Autodesk Fusion 360 part; units mm, degrees
note: some values were not read from the file. Chosen so that the rebuilt part matches the saved one: which pieces of a blend or face edit are solid.
(part 2 of 4)
  circle A222 centre (-225.2664, 136.3493) radius 1.5
  circle A223 centre (-233.5214, 157.9393) radius 0.875
  circle A224 centre (-238.6014, 157.9393) radius 1.9939
  circle A225 centre (-243.6814, 157.9393) radius 0.875
  circle A226 centre (-234.7914, 155.3993) radius 1.5
  circle A227 centre (-241.1414, 152.8593) radius 1.5
  circle A228 centre (-252.5714, 157.9393) radius 0.875
  circle A229 centre (-257.6514, 157.9393) radius 1.9939
  circle A230 centre (-262.7314, 157.9393) radius 0.875
  circle A231 centre (-253.8414, 155.3993) radius 1.5
  circle A232 centre (-260.1914, 152.8593) radius 1.5
  circle A233 centre (-271.6214, 157.9393) radius 0.875
  circle A234 centre (-276.7014, 157.9393) radius 1.9939
  circle A235 centre (-281.7814, 157.9393) radius 0.875
  circle A236 centre (-272.8914, 155.3993) radius 1.5
  circle A237 centre (-279.2414, 152.8593) radius 1.5
  circle A238 centre (-290.6714, 157.9393) radius 0.875
  circle A239 centre (-295.7514, 157.9393) radius 1.9939
  circle A240 centre (-300.8314, 157.9393) radius 0.875
  circle A241 centre (-291.9414, 155.3993) radius 1.5
  circle A242 centre (-298.2914, 152.8593) radius 1.5
  arc A243 (-228.0198, 142.4254) -> (-227.3325, 143.1126) centre (-227.7593, 142.8521) ccw
  arc A244 (-228.0198, 142.4254) -> (-228.1761, 142.4693) centre (-228.176, 142.1696) ccw
  line L196 (-228.1761, 142.4693) -> (-229.0764, 142.4693)
  line L197 (-229.0764, 142.4693) -> (-229.9768, 142.4693)
  arc A245 (-229.9768, 142.4693) -> (-230.1331, 142.4254) centre (-229.9768, 142.1693) ccw
  arc A246 (-230.8204, 143.1126) -> (-230.1331, 142.4254) centre (-230.3936, 142.8521) ccw
  arc A247 (-230.8204, 143.1126) -> (-230.7764, 143.2689) centre (-231.0764, 143.2689) ccw
  line L198 (-230.7764, 143.2689) -> (-230.7764, 143.9693)
  line L199 (-230.7764, 143.9693) -> (-230.7764, 144.6696)
  arc A248 (-230.7764, 144.6696) -> (-230.8204, 144.8259) centre (-231.0764, 144.6696) ccw
  arc A249 (-230.1331, 145.5132) -> (-230.8204, 144.8259) centre (-230.3936, 145.0864) ccw
  arc A250 (-230.1331, 145.5132) -> (-229.9768, 145.4693) centre (-229.9768, 145.7693) ccw
  line L200 (-229.9768, 145.4693) -> (-229.0764, 145.4693)
  line L201 (-229.0764, 145.4693) -> (-228.1761, 145.4693)
  arc A251 (-228.1761, 145.4693) -> (-228.0198, 145.5132) centre (-228.1761, 145.7693) ccw
  arc A252 (-227.3325, 144.8259) -> (-228.0198, 145.5132) centre (-227.7593, 145.0864) ccw
  arc A253 (-227.3325, 144.8259) -> (-227.3764, 144.6696) centre (-227.0764, 144.6696) ccw
  line L202 (-227.3764, 144.6696) -> (-227.3764, 143.9693)
  line L203 (-227.3764, 143.9693) -> (-227.3764, 143.2689)
  arc A254 (-227.3764, 143.2689) -> (-227.3325, 143.1126) centre (-227.0764, 143.2689) ccw
  circle A255 centre (-229.0764, 138.8893) radius 1.9939
  circle A256 centre (-234.1564, 138.8893) radius 0.875
  circle A257 centre (-243.0464, 138.8893) radius 0.875
  arc A258 (-247.0698, 142.4254) -> (-246.3825, 143.1126) centre (-246.8093, 142.8521) ccw
  arc A259 (-247.0698, 142.4254) -> (-247.2261, 142.4693) centre (-247.226, 142.1696) ccw
  line L204 (-247.2261, 142.4693) -> (-248.1264, 142.4693)
  line L205 (-248.1264, 142.4693) -> (-249.0268, 142.4693)
  arc A260 (-249.0268, 142.4693) -> (-249.1831, 142.4254) centre (-249.0268, 142.1693) ccw
  arc A261 (-249.8704, 143.1126) -> (-249.1831, 142.4254) centre (-249.4436, 142.8521) ccw
  arc A262 (-249.8704, 143.1126) -> (-249.8264, 143.2689) centre (-250.1264, 143.2689) ccw
  line L206 (-249.8264, 143.2689) -> (-249.8264, 143.9693)
  line L207 (-249.8264, 143.9693) -> (-249.8264, 144.6696)
  arc A263 (-249.8264, 144.6696) -> (-249.8704, 144.8259) centre (-250.1264, 144.6696) ccw
  arc A264 (-249.1831, 145.5132) -> (-249.8704, 144.8259) centre (-249.4436, 145.0864) ccw
  arc A265 (-249.1831, 145.5132) -> (-249.0268, 145.4693) centre (-249.0268, 145.7693) ccw
  line L208 (-249.0268, 145.4693) -> (-248.1264, 145.4693)
  line L209 (-248.1264, 145.4693) -> (-247.2261, 145.4693)
  arc A266 (-247.2261, 145.4693) -> (-247.0698, 145.5132) centre (-247.2261, 145.7693) ccw
  arc A267 (-246.3825, 144.8259) -> (-247.0698, 145.5132) centre (-246.8093, 145.0864) ccw
  arc A268 (-246.3825, 144.8259) -> (-246.4264, 144.6696) centre (-246.1264, 144.6696) ccw
  line L210 (-246.4264, 144.6696) -> (-246.4264, 143.9693)
  line L211 (-246.4264, 143.9693) -> (-246.4264, 143.2689)
  arc A269 (-246.4264, 143.2689) -> (-246.3825, 143.1126) centre (-246.1264, 143.2689) ccw
  circle A270 centre (-248.1264, 138.8893) radius 1.9939
  circle A271 centre (-253.2064, 138.8893) radius 0.875
  circle A272 centre (-262.0964, 138.8893) radius 0.875
  circle A273 centre (-231.6164, 133.8093) radius 1.5
  circle A274 centre (-244.3164, 136.3493) radius 1.5
  circle A275 centre (-250.6664, 133.8093) radius 1.5
  circle A276 centre (-263.3664, 136.3493) radius 1.5
  arc A277 (-266.1198, 142.4254) -> (-265.4325, 143.1126) centre (-265.8593, 142.8521) ccw
  arc A278 (-266.1198, 142.4254) -> (-266.2761, 142.4693) centre (-266.276, 142.1696) ccw
  line L212 (-266.2761, 142.4693) -> (-267.1764, 142.4693)
  line L213 (-267.1764, 142.4693) -> (-268.0768, 142.4693)
  arc A279 (-268.0768, 142.4693) -> (-268.2331, 142.4254) centre (-268.0768, 142.1693) ccw
  arc A280 (-268.9204, 143.1126) -> (-268.2331, 142.4254) centre (-268.4936, 142.8521) ccw
  arc A281 (-268.9204, 143.1126) -> (-268.8764, 143.2689) centre (-269.1764, 143.2689) ccw
  line L214 (-268.8764, 143.2689) -> (-268.8764, 143.9693)
  line L215 (-268.8764, 143.9693) -> (-268.8764, 144.6696)
  arc A282 (-268.8764, 144.6696) -> (-268.9204, 144.8259) centre (-269.1764, 144.6696) ccw
  arc A283 (-268.2331, 145.5132) -> (-268.9204, 144.8259) centre (-268.4936, 145.0864) ccw
  arc A284 (-268.2331, 145.5132) -> (-268.0768, 145.4693) centre (-268.0768, 145.7693) ccw
  line L216 (-268.0768, 145.4693) -> (-267.1764, 145.4693)
  line L217 (-267.1764, 145.4693) -> (-266.2761, 145.4693)
  arc A285 (-266.2761, 145.4693) -> (-266.1198, 145.5132) centre (-266.2761, 145.7693) ccw
  arc A286 (-265.4325, 144.8259) -> (-266.1198, 145.5132) centre (-265.8593, 145.0864) ccw
  arc A287 (-265.4325, 144.8259) -> (-265.4764, 144.6696) centre (-265.1764, 144.6696) ccw
  line L218 (-265.4764, 144.6696) -> (-265.4764, 143.9693)
  line L219 (-265.4764, 143.9693) -> (-265.4764, 143.2689)
  arc A288 (-265.4764, 143.2689) -> (-265.4325, 143.1126) centre (-265.1764, 143.2689) ccw
  circle A289 centre (-267.1764, 138.8893) radius 1.9939
  circle A290 centre (-272.2564, 138.8893) radius 0.875
  circle A291 centre (-281.1464, 138.8893) radius 0.875
  arc A292 (-287.9704, 143.1126) -> (-287.2831, 142.4254) centre (-287.5436, 142.8521) ccw
  arc A293 (-287.9704, 143.1126) -> (-287.9264, 143.2689) centre (-288.2264, 143.2689) ccw
  line L220 (-287.9264, 143.2689) -> (-287.9264, 143.9693)
  line L221 (-287.9264, 143.9693) -> (-287.9264, 144.6696)
  arc A294 (-287.9264, 144.6696) -> (-287.9704, 144.8259) centre (-288.2264, 144.6696) ccw
  arc A295 (-287.2831, 145.5132) -> (-287.9704, 144.8259) centre (-287.5436, 145.0864) ccw
  arc A296 (-287.2831, 145.5132) -> (-287.1268, 145.4693) centre (-287.1268, 145.7693) ccw
  line L222 (-287.1268, 145.4693) -> (-286.2264, 145.4693)
  line L223 (-286.2264, 145.4693) -> (-285.3261, 145.4693)
  arc A297 (-285.3261, 145.4693) -> (-285.1698, 145.5132) centre (-285.3261, 145.7693) ccw
  arc A298 (-284.4825, 144.8259) -> (-285.1698, 145.5132) centre (-284.9093, 145.0864) ccw
  arc A299 (-284.4825, 144.8259) -> (-284.5264, 144.6696) centre (-284.2264, 144.6696) ccw
  line L224 (-284.5264, 144.6696) -> (-284.5264, 143.9693)
  line L225 (-284.5264, 143.9693) -> (-284.5264, 143.2689)
  arc A300 (-284.5264, 143.2689) -> (-284.4825, 143.1126) centre (-284.2264, 143.2689) ccw
  arc A301 (-285.1698, 142.4254) -> (-284.4825, 143.1126) centre (-284.9093, 142.8521) ccw
  arc A302 (-285.1698, 142.4254) -> (-285.3261, 142.4693) centre (-285.326, 142.1696) ccw
  line L226 (-285.3261, 142.4693) -> (-286.2264, 142.4693)
  line L227 (-286.2264, 142.4693) -> (-287.1268, 142.4693)
  arc A303 (-287.1268, 142.4693) -> (-287.2831, 142.4254) centre (-287.1268, 142.1693) ccw
  arc A304 (-307.0204, 143.1126) -> (-306.3331, 142.4254) centre (-306.5936, 142.8521) ccw
  arc A305 (-307.0204, 143.1126) -> (-306.9764, 143.2689) centre (-307.2764, 143.2689) ccw
  line L228 (-306.9764, 143.2689) -> (-306.9764, 143.9693)
  line L229 (-306.9764, 143.9693) -> (-306.9764, 144.6696)
  arc A306 (-306.9764, 144.6696) -> (-307.0204, 144.8259) centre (-307.2764, 144.6696) ccw
  arc A307 (-306.3331, 145.5132) -> (-307.0204, 144.8259) centre (-306.5936, 145.0864) ccw
  arc A308 (-306.3331, 145.5132) -> (-306.1768, 145.4693) centre (-306.1768, 145.7693) ccw
  line L230 (-306.1768, 145.4693) -> (-305.2764, 145.4693)
  line L231 (-305.2764, 145.4693) -> (-304.3761, 145.4693)
  arc A309 (-304.3761, 145.4693) -> (-304.2198, 145.5132) centre (-304.3761, 145.7693) ccw
  arc A310 (-303.5325, 144.8259) -> (-304.2198, 145.5132) centre (-303.9593, 145.0864) ccw
  arc A311 (-303.5325, 144.8259) -> (-303.5764, 144.6696) centre (-303.2764, 144.6696) ccw
  line L232 (-303.5764, 144.6696) -> (-303.5764, 143.9693)
  line L233 (-303.5764, 143.9693) -> (-303.5764, 143.2689)
  arc A312 (-303.5764, 143.2689) -> (-303.5325, 143.1126) centre (-303.2764, 143.2689) ccw
  arc A313 (-304.2198, 142.4254) -> (-303.5325, 143.1126) centre (-303.9593, 142.8521) ccw
  arc A314 (-304.2198, 142.4254) -> (-304.3761, 142.4693) centre (-304.376, 142.1696) ccw
  line L234 (-304.3761, 142.4693) -> (-305.2764, 142.4693)
  line L235 (-305.2764, 142.4693) -> (-306.1768, 142.4693)
  arc A315 (-306.1768, 142.4693) -> (-306.3331, 142.4254) centre (-306.1768, 142.1693) ccw
  circle A316 centre (-286.2264, 138.8893) radius 1.9939
  circle A317 centre (-291.3064, 138.8893) radius 0.875
  circle A318 centre (-300.1964, 138.8893) radius 0.875
  circle A319 centre (-305.2764, 138.8893) radius 1.9939
  circle A320 centre (-269.7164, 133.8093) radius 1.5
  circle A321 centre (-282.4164, 136.3493) radius 1.5
  circle A322 centre (-288.7664, 133.8093) radius 1.5
  circle A323 centre (-301.4664, 136.3493) radius 1.5
  circle A324 centre (-326.7077, 191.2768) radius 1.1
  circle A325 centre (-343.0589, 176.9893) radius 0.875
  arc A326 (-349.8829, 181.2126) -> (-349.1956, 180.5254) centre (-349.4561, 180.9521) ccw
  arc A327 (-349.8829, 181.2126) -> (-349.8389, 181.3689) centre (-350.1389, 181.3689) ccw
  line L236 (-349.8389, 181.3689) -> (-349.8389, 182.0693)
  line L237 (-349.8389, 182.0693) -> (-349.8389, 182.7696)
  arc A328 (-349.8389, 182.7696) -> (-349.8829, 182.9259) centre (-350.1389, 182.7696) ccw
  arc A329 (-349.1956, 183.6132) -> (-349.8829, 182.9259) centre (-349.4561, 183.1864) ccw
  arc A330 (-349.1956, 183.6132) -> (-349.0393, 183.5693) centre (-349.0393, 183.8693) ccw
  line L238 (-349.0393, 183.5693) -> (-348.1389, 183.5693)
  line L239 (-348.1389, 183.5693) -> (-347.2386, 183.5693)
  arc A331 (-347.2386, 183.5693) -> (-347.0823, 183.6132) centre (-347.2386, 183.8693) ccw
  arc A332 (-346.395, 182.9259) -> (-347.0823, 183.6132) centre (-346.8218, 183.1864) ccw
  arc A333 (-346.395, 182.9259) -> (-346.4389, 182.7696) centre (-346.1389, 182.7696) ccw
  line L240 (-346.4389, 182.7696) -> (-346.4389, 182.0693)
  line L241 (-346.4389, 182.0693) -> (-346.4389, 181.3689)
  arc A334 (-346.4389, 181.3689) -> (-346.395, 181.2126) centre (-346.1389, 181.3689) ccw
  arc A335 (-347.0823, 180.5254) -> (-346.395, 181.2126) centre (-346.8218, 180.9521) ccw
  arc A336 (-347.0823, 180.5254) -> (-347.2386, 180.5693) centre (-347.2385, 180.2696) ccw
  line L242 (-347.2386, 180.5693) -> (-348.1389, 180.5693)
  line L243 (-348.1389, 180.5693) -> (-349.0393, 180.5693)
  arc A337 (-349.0393, 180.5693) -> (-349.1956, 180.5254) centre (-349.0393, 180.2693) ccw
  circle A338 centre (-348.1389, 176.9893) radius 1.9939
  circle A339 centre (-353.2189, 176.9893) radius 0.875
  circle A340 centre (-362.1089, 176.9893) radius 0.875
  arc A341 (-368.9329, 181.2126) -> (-368.2456, 180.5254) centre (-368.5061, 180.9521) ccw
  arc A342 (-368.9329, 181.2126) -> (-368.8889, 181.3689) centre (-369.1889, 181.3689) ccw
  line L244 (-368.8889, 181.3689) -> (-368.8889, 182.0693)
  line L245 (-368.8889, 182.0693) -> (-368.8889, 182.7696)
  arc A343 (-368.8889, 182.7696) -> (-368.9329, 182.9259) centre (-369.1889, 182.7696) ccw
  arc A344 (-368.2456, 183.6132) -> (-368.9329, 182.9259) centre (-368.5061, 183.1864) ccw
  arc A345 (-368.2456, 183.6132) -> (-368.0893, 183.5693) centre (-368.0893, 183.8693) ccw
  line L246 (-368.0893, 183.5693) -> (-367.1889, 183.5693)
  line L247 (-367.1889, 183.5693) -> (-366.2886, 183.5693)
  arc A346 (-366.2886, 183.5693) -> (-366.1323, 183.6132) centre (-366.2886, 183.8693) ccw
  arc A347 (-365.445, 182.9259) -> (-366.1323, 183.6132) centre (-365.8718, 183.1864) ccw
  arc A348 (-365.445, 182.9259) -> (-365.4889, 182.7696) centre (-365.1889, 182.7696) ccw
  line L248 (-365.4889, 182.7696) -> (-365.4889, 182.0693)
  line L249 (-365.4889, 182.0693) -> (-365.4889, 181.3689)
  arc A349 (-365.4889, 181.3689) -> (-365.445, 181.2126) centre (-365.1889, 181.3689) ccw
  arc A350 (-366.1323, 180.5254) -> (-365.445, 181.2126) centre (-365.8718, 180.9521) ccw
  arc A351 (-366.1323, 180.5254) -> (-366.2886, 180.5693) centre (-366.2885, 180.2696) ccw
  line L250 (-366.2886, 180.5693) -> (-367.1889, 180.5693)
  line L251 (-367.1889, 180.5693) -> (-368.0893, 180.5693)
  arc A352 (-368.0893, 180.5693) -> (-368.2456, 180.5254) centre (-368.0893, 180.2693) ccw
  circle A353 centre (-367.1889, 176.9893) radius 1.9939
  circle A354 centre (-372.2689, 176.9893) radius 0.875
  circle A355 centre (-381.1589, 176.9893) radius 0.875
  circle A356 centre (-344.3289, 174.4493) radius 1.5
  arc A357 (-316.5454, 162.1626) -> (-315.8581, 161.4754) centre (-316.1186, 161.9021) ccw
  arc A358 (-316.5454, 162.1626) -> (-316.5014, 162.3189) centre (-316.8014, 162.3189) ccw
  line L252 (-316.5014, 162.3189) -> (-316.5014, 163.0193)
  line L253 (-316.5014, 163.0193) -> (-316.5014, 163.7196)
  arc A359 (-316.5014, 163.7196) -> (-316.5454, 163.8759) centre (-316.8014, 163.7196) ccw
  arc A360 (-315.8581, 164.5632) -> (-316.5454, 163.8759) centre (-316.1186, 164.1364) ccw
  arc A361 (-315.8581, 164.5632) -> (-315.7018, 164.5193) centre (-315.7018, 164.8193) ccw
  line L254 (-315.7018, 164.5193) -> (-314.8014, 164.5193)
  line L255 (-314.8014, 164.5193) -> (-313.9011, 164.5193)
  arc A362 (-313.9011, 164.5193) -> (-313.7448, 164.5632) centre (-313.9011, 164.8193) ccw
  arc A363 (-313.0575, 163.8759) -> (-313.7448, 164.5632) centre (-313.4843, 164.1364) ccw
  arc A364 (-313.0575, 163.8759) -> (-313.1014, 163.7196) centre (-312.8014, 163.7196) ccw
  line L256 (-313.1014, 163.7196) -> (-313.1014, 163.0193)
  line L257 (-313.1014, 163.0193) -> (-313.1014, 162.3189)
  arc A365 (-313.1014, 162.3189) -> (-313.0575, 162.1626) centre (-312.8014, 162.3189) ccw
  arc A366 (-313.7448, 161.4754) -> (-313.0575, 162.1626) centre (-313.4843, 161.9021) ccw
  arc A367 (-313.7448, 161.4754) -> (-313.9011, 161.5193) centre (-313.901, 161.2196) ccw
  line L258 (-313.9011, 161.5193) -> (-314.8014, 161.5193)
  line L259 (-314.8014, 161.5193) -> (-315.7018, 161.5193)
  arc A368 (-315.7018, 161.5193) -> (-315.8581, 161.4754) centre (-315.7018, 161.2193) ccw
  arc A369 (-335.5954, 162.1626) -> (-334.9081, 161.4754) centre (-335.1686, 161.9021) ccw
  arc A370 (-335.5954, 162.1626) -> (-335.5514, 162.3189) centre (-335.8514, 162.3189) ccw
  line L260 (-335.5514, 162.3189) -> (-335.5514, 163.0193)
  line L261 (-335.5514, 163.0193) -> (-335.5514, 163.7196)
  arc A371 (-335.5514, 163.7196) -> (-335.5954, 163.8759) centre (-335.8514, 163.7196) ccw
  arc A372 (-334.9081, 164.5632) -> (-335.5954, 163.8759) centre (-335.1686, 164.1364) ccw
  arc A373 (-334.9081, 164.5632) -> (-334.7518, 164.5193) centre (-334.7518, 164.8193) ccw
  line L262 (-334.7518, 164.5193) -> (-333.8514, 164.5193)
  line L263 (-333.8514, 164.5193) -> (-332.9511, 164.5193)
  arc A374 (-332.9511, 164.5193) -> (-332.7948, 164.5632) centre (-332.9511, 164.8193) ccw
  arc A375 (-332.1075, 163.8759) -> (-332.7948, 164.5632) centre (-332.5343, 164.1364) ccw
  arc A376 (-332.1075, 163.8759) -> (-332.1514, 163.7196) centre (-331.8514, 163.7196) ccw
  line L264 (-332.1514, 163.7196) -> (-332.1514, 163.0193)
  line L265 (-332.1514, 163.0193) -> (-332.1514, 162.3189)
  arc A377 (-332.1514, 162.3189) -> (-332.1075, 162.1626) centre (-331.8514, 162.3189) ccw
  arc A378 (-332.7948, 161.4754) -> (-332.1075, 162.1626) centre (-332.5343, 161.9021) ccw
  arc A379 (-332.7948, 161.4754) -> (-332.9511, 161.5193) centre (-332.951, 161.2196) ccw
  line L266 (-332.9511, 161.5193) -> (-333.8514, 161.5193)
  line L267 (-333.8514, 161.5193) -> (-334.7518, 161.5193)
  arc A380 (-334.7518, 161.5193) -> (-334.9081, 161.4754) centre (-334.7518, 161.2193) ccw
  circle A381 centre (-363.3789, 174.4493) radius 1.5
  circle A382 centre (-350.6789, 171.9093) radius 1.5
  circle A383 centre (-382.4289, 174.4493) radius 1.5
  circle A384 centre (-369.7289, 171.9093) radius 1.5
  arc A385 (-354.6454, 162.1626) -> (-353.9581, 161.4754) centre (-354.2186, 161.9021) ccw
  arc A386 (-354.6454, 162.1626) -> (-354.6014, 162.3189) centre (-354.9014, 162.3189) ccw
  line L268 (-354.6014, 162.3189) -> (-354.6014, 163.0193)
  line L269 (-354.6014, 163.0193) -> (-354.6014, 163.7196)
  arc A387 (-354.6014, 163.7196) -> (-354.6454, 163.8759) centre (-354.9014, 163.7196) ccw
  arc A388 (-353.9581, 164.5632) -> (-354.6454, 163.8759) centre (-354.2186, 164.1364) ccw
  arc A389 (-353.9581, 164.5632) -> (-353.8018, 164.5193) centre (-353.8018, 164.8193) ccw
  line L270 (-353.8018, 164.5193) -> (-352.9014, 164.5193)
  line L271 (-352.9014, 164.5193) -> (-352.0011, 164.5193)
  arc A390 (-352.0011, 164.5193) -> (-351.8448, 164.5632) centre (-352.0011, 164.8193) ccw
  arc A391 (-351.1575, 163.8759) -> (-351.8448, 164.5632) centre (-351.5843, 164.1364) ccw
  arc A392 (-351.1575, 163.8759) -> (-351.2014, 163.7196) centre (-350.9014, 163.7196) ccw
  line L272 (-351.2014, 163.7196) -> (-351.2014, 163.0193)
  line L273 (-351.2014, 163.0193) -> (-351.2014, 162.3189)
  arc A393 (-351.2014, 162.3189) -> (-351.1575, 162.1626) centre (-350.9014, 162.3189) ccw
  arc A394 (-351.8448, 161.4754) -> (-351.1575, 162.1626) centre (-351.5843, 161.9021) ccw
  arc A395 (-351.8448, 161.4754) -> (-352.0011, 161.5193) centre (-352.001, 161.2196) ccw
  line L274 (-352.0011, 161.5193) -> (-352.9014, 161.5193)
  line L275 (-352.9014, 161.5193) -> (-353.8018, 161.5193)
  arc A396 (-353.8018, 161.5193) -> (-353.9581, 161.4754) centre (-353.8018, 161.2193) ccw
  arc A397 (-373.6954, 162.1626) -> (-373.0081, 161.4754) centre (-373.2686, 161.9021) ccw
  arc A398 (-373.6954, 162.1626) -> (-373.6514, 162.3189) centre (-373.9514, 162.3189) ccw
  line L276 (-373.6514, 162.3189) -> (-373.6514, 163.0193)
  line L277 (-373.6514, 163.0193) -> (-373.6514, 163.7196)
  arc A399 (-373.6514, 163.7196) -> (-373.6954, 163.8759) centre (-373.9514, 163.7196) ccw
  arc A400 (-373.0081, 164.5632) -> (-373.6954, 163.8759) centre (-373.2686, 164.1364) ccw
  arc A401 (-373.0081, 164.5632) -> (-372.8518, 164.5193) centre (-372.8518, 164.8193) ccw
  line L278 (-372.8518, 164.5193) -> (-371.9514, 164.5193)
  line L279 (-371.9514, 164.5193) -> (-371.0511, 164.5193)
  arc A402 (-371.0511, 164.5193) -> (-370.8948, 164.5632) centre (-371.0511, 164.8193) ccw
  arc A403 (-370.2075, 163.8759) -> (-370.8948, 164.5632) centre (-370.6343, 164.1364) ccw
  arc A404 (-370.2075, 163.8759) -> (-370.2514, 163.7196) centre (-369.9514, 163.7196) ccw
  line L280 (-370.2514, 163.7196) -> (-370.2514, 163.0193)
  line L281 (-370.2514, 163.0193) -> (-370.2514, 162.3189)
  arc A405 (-370.2514, 162.3189) -> (-370.2075, 162.1626) centre (-369.9514, 162.3189) ccw
  arc A406 (-370.8948, 161.4754) -> (-370.2075, 162.1626) centre (-370.6343, 161.9021) ccw
  arc A407 (-370.8948, 161.4754) -> (-371.0511, 161.5193) centre (-371.051, 161.2196) ccw
  line L282 (-371.0511, 161.5193) -> (-371.9514, 161.5193)
  line L283 (-371.9514, 161.5193) -> (-372.8518, 161.5193)
  arc A408 (-372.8518, 161.5193) -> (-373.0081, 161.4754) centre (-372.8518, 161.2193) ccw
  arc A409 (-411.7954, 185.9751) -> (-411.1081, 185.2879) centre (-411.3686, 185.7146) ccw
  arc A410 (-411.7954, 185.9751) -> (-411.7514, 186.1314) centre (-412.0514, 186.1314) ccw
  line L284 (-411.7514, 186.1314) -> (-411.7514, 186.8318)
  line L285 (-411.7514, 186.8318) -> (-411.7514, 187.5321)
  arc A411 (-411.7514, 187.5321) -> (-411.7954, 187.6884) centre (-412.0514, 187.5321) ccw
  arc A412 (-411.1081, 188.3757) -> (-411.7954, 187.6884) centre (-411.3686, 187.9489) ccw
  arc A413 (-411.1081, 188.3757) -> (-410.9518, 188.3318) centre (-410.9518, 188.6318) ccw
  line L286 (-410.9518, 188.3318) -> (-410.0514, 188.3318)
  line L287 (-410.0514, 188.3318) -> (-409.1511, 188.3318)
  arc A414 (-409.1511, 188.3318) -> (-408.9948, 188.3757) centre (-409.1511, 188.6318) ccw
  arc A415 (-408.3075, 187.6884) -> (-408.9948, 188.3757) centre (-408.7343, 187.9489) ccw
  arc A416 (-408.3075, 187.6884) -> (-408.3514, 187.5321) centre (-408.0514, 187.5321) ccw
  line L288 (-408.3514, 187.5321) -> (-408.3514, 186.8318)
  line L289 (-408.3514, 186.8318) -> (-408.3514, 186.1314)
  arc A417 (-408.3514, 186.1314) -> (-408.3075, 185.9751) centre (-408.0514, 186.1314) ccw
  arc A418 (-408.9948, 185.2879) -> (-408.3075, 185.9751) centre (-408.7343, 185.7146) ccw
  arc A419 (-408.9948, 185.2879) -> (-409.1511, 185.3318) centre (-409.151, 185.0321) ccw
  line L290 (-409.1511, 185.3318) -> (-410.0514, 185.3318)
  line L291 (-410.0514, 185.3318) -> (-410.9518, 185.3318)
  arc A420 (-410.9518, 185.3318) -> (-411.1081, 185.2879) centre (-410.9518, 185.0318) ccw
  arc A421 (-387.9829, 181.2126) -> (-387.2956, 180.5254) centre (-387.5561, 180.9521) ccw
  arc A422 (-387.9829, 181.2126) -> (-387.9389, 181.3689) centre (-388.2389, 181.3689) ccw
  line L292 (-387.9389, 181.3689) -> (-387.9389, 182.0693)
  line L293 (-387.9389, 182.0693) -> (-387.9389, 182.7696)
  arc A423 (-387.9389, 182.7696) -> (-387.9829, 182.9259) centre (-388.2389, 182.7696) ccw
  arc A424 (-387.2956, 183.6132) -> (-387.9829, 182.9259) centre (-387.5561, 183.1864) ccw
  arc A425 (-387.2956, 183.6132) -> (-387.1393, 183.5693) centre (-387.1393, 183.8693) ccw
  line L294 (-387.1393, 183.5693) -> (-386.2389, 183.5693)
  line L295 (-386.2389, 183.5693) -> (-385.3386, 183.5693)
  arc A426 (-385.3386, 183.5693) -> (-385.1823, 183.6132) centre (-385.3386, 183.8693) ccw
  arc A427 (-384.495, 182.9259) -> (-385.1823, 183.6132) centre (-384.9218, 183.1864) ccw
  arc A428 (-384.495, 182.9259) -> (-384.5389, 182.7696) centre (-384.2389, 182.7696) ccw
  line L296 (-384.5389, 182.7696) -> (-384.5389, 182.0693)
  line L297 (-384.5389, 182.0693) -> (-384.5389, 181.3689)
  arc A429 (-384.5389, 181.3689) -> (-384.495, 181.2126) centre (-384.2389, 181.3689) ccw
  arc A430 (-385.1823, 180.5254) -> (-384.495, 181.2126) centre (-384.9218, 180.9521) ccw
  arc A431 (-385.1823, 180.5254) -> (-385.3386, 180.5693) centre (-385.3385, 180.2696) ccw
  line L298 (-385.3386, 180.5693) -> (-386.2389, 180.5693)
  line L299 (-386.2389, 180.5693) -> (-387.1393, 180.5693)
  arc A432 (-387.1393, 180.5693) -> (-387.2956, 180.5254) centre (-387.1393, 180.2693) ccw
  circle A433 centre (-386.2389, 176.9893) radius 1.9939
  circle A434 centre (-391.3189, 176.9893) radius 0.875
  circle A435 centre (-404.9714, 181.7518) radius 0.875
  circle A436 centre (-410.0514, 181.7518) radius 1.9939
  circle A437 centre (-415.1314, 181.7518) radius 0.875
  circle A438 centre (-406.2414, 179.2118) radius 1.5
  circle A439 centre (-412.5914, 176.6718) radius 1.5
  arc A440 (-430.8454, 185.9751) -> (-430.1581, 185.2879) centre (-430.4186, 185.7146) ccw
  arc A441 (-430.8454, 185.9751) -> (-430.8014, 186.1314) centre (-431.1014, 186.1314) ccw
  line L300 (-430.8014, 186.1314) -> (-430.8014, 186.8318)
  line L301 (-430.8014, 186.8318) -> (-430.8014, 187.5321)
  arc A442 (-430.8014, 187.5321) -> (-430.8454, 187.6884) centre (-431.1014, 187.5321) ccw
  arc A443 (-430.1581, 188.3757) -> (-430.8454, 187.6884) centre (-430.4186, 187.9489) ccw
  arc A444 (-430.1581, 188.3757) -> (-430.0018, 188.3318) centre (-430.0018, 188.6318) ccw
  line L302 (-430.0018, 188.3318) -> (-429.1014, 188.3318)
  line L303 (-429.1014, 188.3318) -> (-428.2011, 188.3318)
  arc A445 (-428.2011, 188.3318) -> (-428.0448, 188.3757) centre (-428.2011, 188.6318) ccw
  arc A446 (-427.3575, 187.6884) -> (-428.0448, 188.3757) centre (-427.7843, 187.9489) ccw
  arc A447 (-427.3575, 187.6884) -> (-427.4014, 187.5321) centre (-427.1014, 187.5321) ccw
  line L304 (-427.4014, 187.5321) -> (-427.4014, 186.8318)
  line L305 (-427.4014, 186.8318) -> (-427.4014, 186.1314)
  arc A448 (-427.4014, 186.1314) -> (-427.3575, 185.9751) centre (-427.1014, 186.1314) ccw
  arc A449 (-428.0448, 185.2879) -> (-427.3575, 185.9751) centre (-427.7843, 185.7146) ccw
  arc A450 (-428.0448, 185.2879) -> (-428.2011, 185.3318) centre (-428.201, 185.0321) ccw
  line L306 (-428.2011, 185.3318) -> (-429.1014, 185.3318)
  line L307 (-429.1014, 185.3318) -> (-430.0018, 185.3318)
  arc A451 (-430.0018, 185.3318) -> (-430.1581, 185.2879) centre (-430.0018, 185.0318) ccw
  circle A452 centre (-462.4389, 191.2768) radius 1.1
  arc A453 (-449.8954, 185.9751) -> (-449.2081, 185.2879) centre (-449.4686, 185.7146) ccw
  arc A454 (-449.8954, 185.9751) -> (-449.8514, 186.1314) centre (-450.1514, 186.1314) ccw
  line L308 (-449.8514, 186.1314) -> (-449.8514, 186.8318)
  line L309 (-449.8514, 186.8318) -> (-449.8514, 187.5321)
  arc A455 (-449.8514, 187.5321) -> (-449.8954, 187.6884) centre (-450.1514, 187.5321) ccw
  arc A456 (-449.2081, 188.3757) -> (-449.8954, 187.6884) centre (-449.4686, 187.9489) ccw
  arc A457 (-449.2081, 188.3757) -> (-449.0518, 188.3318) centre (-449.0518, 188.6318) ccw
  line L310 (-449.0518, 188.3318) -> (-448.1514, 188.3318)
  line L311 (-448.1514, 188.3318) -> (-447.2511, 188.3318)
  arc A458 (-447.2511, 188.3318) -> (-447.0948, 188.3757) centre (-447.2511, 188.6318) ccw
  arc A459 (-446.4075, 187.6884) -> (-447.0948, 188.3757) centre (-446.8343, 187.9489) ccw
  arc A460 (-446.4075, 187.6884) -> (-446.4514, 187.5321) centre (-446.1514, 187.5321) ccw
  line L312 (-446.4514, 187.5321) -> (-446.4514, 186.8318)
  line L313 (-446.4514, 186.8318) -> (-446.4514, 186.1314)
  arc A461 (-446.4514, 186.1314) -> (-446.4075, 185.9751) centre (-446.1514, 186.1314) ccw
  arc A462 (-447.0948, 185.2879) -> (-446.4075, 185.9751) centre (-446.8343, 185.7146) ccw
  arc A463 (-447.0948, 185.2879) -> (-447.2511, 185.3318) centre (-447.251, 185.0321) ccw
  line L314 (-447.2511, 185.3318) -> (-448.1514, 185.3318)
  line L315 (-448.1514, 185.3318) -> (-449.0518, 185.3318)
  arc A464 (-449.0518, 185.3318) -> (-449.2081, 185.2879) centre (-449.0518, 185.0318) ccw
  circle A465 centre (-424.0214, 181.7518) radius 0.875
  circle A466 centre (-429.1014, 181.7518) radius 1.9939
  circle A467 centre (-434.1814, 181.7518) radius 0.875
  circle A468 centre (-443.0714, 181.7518) radius 0.875
  circle A469 centre (-425.2914, 179.2118) radius 1.5
  circle A470 centre (-431.6414, 176.6718) radius 1.5
  circle A471 centre (-448.1514, 181.7518) radius 1.9939
  circle A472 centre (-453.2314, 181.7518) radius 0.875
  circle A473 centre (-444.3414, 179.2118) radius 1.5
  circle A474 centre (-450.6914, 176.6718) radius 1.5
  circle A475 centre (-388.7789, 171.9093) radius 1.5
  arc A476 (-399.5454, 162.1626) -> (-398.8581, 161.4754) centre (-399.1186, 161.9021) ccw
  arc A477 (-399.5454, 162.1626) -> (-399.5014, 162.3189) centre (-399.8014, 162.3189) ccw
  line L316 (-399.5014, 162.3189) -> (-399.5014, 163.0193)
  line L317 (-399.5014, 163.0193) -> (-399.5014, 163.7196)
  arc A478 (-399.5014, 163.7196) -> (-399.5454, 163.8759) centre (-399.8014, 163.7196) ccw
  arc A479 (-398.8581, 164.5632) -> (-399.5454, 163.8759) centre (-399.1186, 164.1364) ccw
  arc A480 (-398.8581, 164.5632) -> (-398.7018, 164.5193) centre (-398.7018, 164.8193) ccw
  line L318 (-398.7018, 164.5193) -> (-397.8014, 164.5193)
  line L319 (-397.8014, 164.5193) -> (-396.9011, 164.5193)
  arc A481 (-396.9011, 164.5193) -> (-396.7448, 164.5632) centre (-396.9011, 164.8193) ccw
  arc A482 (-396.0575, 163.8759) -> (-396.7448, 164.5632) centre (-396.4843, 164.1364) ccw
  arc A483 (-396.0575, 163.8759) -> (-396.1014, 163.7196) centre (-395.8014, 163.7196) ccw
  line L320 (-396.1014, 163.7196) -> (-396.1014, 163.0193)
  line L321 (-396.1014, 163.0193) -> (-396.1014, 162.3189)
  arc A484 (-396.1014, 162.3189) -> (-396.0575, 162.1626) centre (-395.8014, 162.3189) ccw
  arc A485 (-396.7448, 161.4754) -> (-396.0575, 162.1626) centre (-396.4843, 161.9021) ccw
  arc A486 (-396.7448, 161.4754) -> (-396.9011, 161.5193) centre (-396.901, 161.2196) ccw
  line L322 (-396.9011, 161.5193) -> (-397.8014, 161.5193)
  line L323 (-397.8014, 161.5193) -> (-398.7018, 161.5193)
  arc A487 (-398.7018, 161.5193) -> (-398.8581, 161.4754) centre (-398.7018, 161.2193) ccw
  arc A488 (-430.8454, 166.9251) -> (-430.1581, 166.2379) centre (-430.4186, 166.6646) ccw
  arc A489 (-430.8454, 166.9251) -> (-430.8014, 167.0814) centre (-431.1014, 167.0814) ccw
  line L324 (-430.8014, 167.0814) -> (-430.8014, 167.7818)
  line L325 (-430.8014, 167.7818) -> (-430.8014, 168.4821)
  arc A490 (-430.8014, 168.4821) -> (-430.8454, 168.6384) centre (-431.1014, 168.4821) ccw
  arc A491 (-430.1581, 169.3257) -> (-430.8454, 168.6384) centre (-430.4186, 168.8989) ccw
  arc A492 (-430.1581, 169.3257) -> (-430.0018, 169.2818) centre (-430.0018, 169.5818) ccw
  line L326 (-430.0018, 169.2818) -> (-429.1014, 169.2818)
  line L327 (-429.1014, 169.2818) -> (-428.2011, 169.2818)
  arc A493 (-428.2011, 169.2818) -> (-428.0448, 169.3257) centre (-428.2011, 169.5818) ccw
  arc A494 (-427.3575, 168.6384) -> (-428.0448, 169.3257) centre (-427.7843, 168.8989) ccw
  arc A495 (-427.3575, 168.6384) -> (-427.4014, 168.4821) centre (-427.1014, 168.4821) ccw
  line L328 (-427.4014, 168.4821) -> (-427.4014, 167.7818)
  line L329 (-427.4014, 167.7818) -> (-427.4014, 167.0814)
  arc A496 (-427.4014, 167.0814) -> (-427.3575, 166.9251) centre (-427.1014, 167.0814) ccw
  arc A497 (-428.0448, 166.2379) -> (-427.3575, 166.9251) centre (-427.7843, 166.6646) ccw
  arc A498 (-428.0448, 166.2379) -> (-428.2011, 166.2818) centre (-428.201, 165.9821) ccw
  line L330 (-428.2011, 166.2818) -> (-429.1014, 166.2818)
  line L331 (-429.1014, 166.2818) -> (-430.0018, 166.2818)
  arc A499 (-430.0018, 166.2818) -> (-430.1581, 166.2379) centre (-430.0018, 165.9818) ccw
  circle A500 centre (-424.0214, 162.7018) radius 0.875
  circle A501 centre (-429.1014, 162.7018) radius 1.9939
  circle A502 centre (-434.1814, 162.7018) radius 0.875
  arc A503 (-454.6579, 162.1626) -> (-453.9706, 161.4754) centre (-454.2311, 161.9021) ccw
  arc A504 (-454.6579, 162.1626) -> (-454.6139, 162.3189) centre (-454.9139, 162.3189) ccw
  line L332 (-454.6139, 162.3189) -> (-454.6139, 163.0193)
  line L333 (-454.6139, 163.0193) -> (-454.6139, 163.7196)
  arc A505 (-454.6139, 163.7196) -> (-454.6579, 163.8759) centre (-454.9139, 163.7196) ccw
  arc A506 (-453.9706, 164.5632) -> (-454.6579, 163.8759) centre (-454.2311, 164.1364) ccw
  arc A507 (-453.9706, 164.5632) -> (-453.8143, 164.5193) centre (-453.8143, 164.8193) ccw
  line L334 (-453.8143, 164.5193) -> (-452.9139, 164.5193)
  line L335 (-452.9139, 164.5193) -> (-452.0136, 164.5193)
  arc A508 (-452.0136, 164.5193) -> (-451.8573, 164.5632) centre (-452.0136, 164.8193) ccw
  arc A509 (-451.17, 163.8759) -> (-451.8573, 164.5632) centre (-451.5968, 164.1364) ccw
  arc A510 (-451.17, 163.8759) -> (-451.2139, 163.7196) centre (-450.9139, 163.7196) ccw
  line L336 (-451.2139, 163.7196) -> (-451.2139, 163.0193)
  line L337 (-451.2139, 163.0193) -> (-451.2139, 162.3189)
  arc A511 (-451.2139, 162.3189) -> (-451.17, 162.1626) centre (-450.9139, 162.3189) ccw
  arc A512 (-451.8573, 161.4754) -> (-451.17, 162.1626) centre (-451.5968, 161.9021) ccw
  arc A513 (-451.8573, 161.4754) -> (-452.0136, 161.5193) centre (-452.0135, 161.2196) ccw
  line L338 (-452.0136, 161.5193) -> (-452.9139, 161.5193)
  line L339 (-452.9139, 161.5193) -> (-453.8143, 161.5193)
  arc A514 (-453.8143, 161.5193) -> (-453.9706, 161.4754) centre (-453.8143, 161.2193) ccw
  circle A515 centre (-309.7214, 157.9393) radius 0.875
  circle A516 centre (-314.8014, 157.9393) radius 1.9939
  circle A517 centre (-319.8814, 157.9393) radius 0.875
  circle A518 centre (-310.9914, 155.3993) radius 1.5
  circle A519 centre (-317.3414, 152.8593) radius 1.5
  circle A520 centre (-328.7714, 157.9393) radius 0.875
  circle A521 centre (-333.8514, 157.9393) radius 1.9939
  circle A522 centre (-338.9314, 157.9393) radius 0.875
  circle A523 centre (-330.0414, 155.3993) radius 1.5
  circle A524 centre (-336.3914, 152.8593) radius 1.5
  circle A525 centre (-347.8214, 157.9393) radius 0.875
  circle A526 centre (-352.9014, 157.9393) radius 1.9939
  circle A527 centre (-357.9814, 157.9393) radius 0.875
  circle A528 centre (-349.0914, 155.3993) radius 1.5
  circle A529 centre (-355.4414, 152.8593) radius 1.5
  circle A530 centre (-366.8714, 157.9393) radius 0.875
  circle A531 centre (-371.9514, 157.9393) radius 1.9939
  circle A532 centre (-377.0314, 157.9393) radius 0.875
  circle A533 centre (-368.1414, 155.3993) radius 1.5
  circle A534 centre (-374.4914, 152.8593) radius 1.5
  arc A535 (-326.0704, 143.1126) -> (-325.3831, 142.4254) centre (-325.6436, 142.8521) ccw
  arc A536 (-326.0704, 143.1126) -> (-326.0264, 143.2689) centre (-326.3264, 143.2689) ccw
  line L340 (-326.0264, 143.2689) -> (-326.0264, 143.9693)
  line L341 (-326.0264, 143.9693) -> (-326.0264, 144.6696)
  arc A537 (-326.0264, 144.6696) -> (-326.0704, 144.8259) centre (-326.3264, 144.6696) ccw
  arc A538 (-325.3831, 145.5132) -> (-326.0704, 144.8259) centre (-325.6436, 145.0864) ccw
  arc A539 (-325.3831, 145.5132) -> (-325.2268, 145.4693) centre (-325.2268, 145.7693) ccw
  line L342 (-325.2268, 145.4693) -> (-324.3264, 145.4693)
  line L343 (-324.3264, 145.4693) -> (-323.4261, 145.4693)
  arc A540 (-323.4261, 145.4693) -> (-323.2698, 145.5132) centre (-323.4261, 145.7693) ccw
  arc A541 (-322.5825, 144.8259) -> (-323.2698, 145.5132) centre (-323.0093, 145.0864) ccw
  arc A542 (-322.5825, 144.8259) -> (-322.6264, 144.6696) centre (-322.3264, 144.6696) ccw
  line L344 (-322.6264, 144.6696) -> (-322.6264, 143.9693)
  line L345 (-322.6264, 143.9693) -> (-322.6264, 143.2689)
  arc A543 (-322.6264, 143.2689) -> (-322.5825, 143.1126) centre (-322.3264, 143.2689) ccw
  arc A544 (-323.2698, 142.4254) -> (-322.5825, 143.1126) centre (-323.0093, 142.8521) ccw
  arc A545 (-323.2698, 142.4254) -> (-323.4261, 142.4693) centre (-323.426, 142.1696) ccw
  line L346 (-323.4261, 142.4693) -> (-324.3264, 142.4693)
  line L347 (-324.3264, 142.4693) -> (-325.2268, 142.4693)
  arc A546 (-325.2268, 142.4693) -> (-325.3831, 142.4254) centre (-325.2268, 142.1693) ccw
  circle A547 centre (-310.3564, 138.8893) radius 0.875
  circle A548 centre (-319.2464, 138.8893) radius 0.875
  circle A549 centre (-324.3264, 138.8893) radius 1.9939
  arc A550 (-345.1204, 143.1126) -> (-344.4331, 142.4254) centre (-344.6936, 142.8521) ccw
  arc A551 (-345.1204, 143.1126) -> (-345.0764, 143.2689) centre (-345.3764, 143.2689) ccw
  line L348 (-345.0764, 143.2689) -> (-345.0764, 143.9693)
  line L349 (-345.0764, 143.9693) -> (-345.0764, 144.6696)
  arc A552 (-345.0764, 144.6696) -> (-345.1204, 144.8259) centre (-345.3764, 144.6696) ccw
  arc A553 (-344.4331, 145.5132) -> (-345.1204, 144.8259) centre (-344.6936, 145.0864) ccw
  arc A554 (-344.4331, 145.5132) -> (-344.2768, 145.4693) centre (-344.2768, 145.7693) ccw
  line L350 (-344.2768, 145.4693) -> (-343.3764, 145.4693)
  line L351 (-343.3764, 145.4693) -> (-342.4761, 145.4693)
  arc A555 (-342.4761, 145.4693) -> (-342.3198, 145.5132) centre (-342.4761, 145.7693) ccw
  arc A556 (-341.6325, 144.8259) -> (-342.3198, 145.5132) centre (-342.0593, 145.0864) ccw
  arc A557 (-341.6325, 144.8259) -> (-341.6764, 144.6696) centre (-341.3764, 144.6696) ccw
  line L352 (-341.6764, 144.6696) -> (-341.6764, 143.9693)
  line L353 (-341.6764, 143.9693) -> (-341.6764, 143.2689)
  arc A558 (-341.6764, 143.2689) -> (-341.6325, 143.1126) centre (-341.3764, 143.2689) ccw
  arc A559 (-342.3198, 142.4254) -> (-341.6325, 143.1126) centre (-342.0593, 142.8521) ccw
  arc A560 (-342.3198, 142.4254) -> (-342.4761, 142.4693) centre (-342.476, 142.1696) ccw
  line L354 (-342.4761, 142.4693) -> (-343.3764, 142.4693)
  line L355 (-343.3764, 142.4693) -> (-344.2768, 142.4693)
  arc A561 (-344.2768, 142.4693) -> (-344.4331, 142.4254) centre (-344.2768, 142.1693) ccw
  circle A562 centre (-329.4064, 138.8893) radius 0.875
  circle A563 centre (-338.2964, 138.8893) radius 0.875
  circle A564 centre (-343.3764, 138.8893) radius 1.9939
  circle A565 centre (-307.8164, 133.8093) radius 1.5
  circle A566 centre (-320.5164, 136.3493) radius 1.5
  circle A567 centre (-326.8664, 133.8093) radius 1.5
  circle A568 centre (-339.5664, 136.3493) radius 1.5
  arc A569 (-364.1704, 143.1126) -> (-363.4831, 142.4254) centre (-363.7436, 142.8521) ccw
  arc A570 (-364.1704, 143.1126) -> (-364.1264, 143.2689) centre (-364.4264, 143.2689) ccw
  line L356 (-364.1264, 143.2689) -> (-364.1264, 143.9693)
  line L357 (-364.1264, 143.9693) -> (-364.1264, 144.6696)
  arc A571 (-364.1264, 144.6696) -> (-364.1704, 144.8259) centre (-364.4264, 144.6696) ccw
  arc A572 (-363.4831, 145.5132) -> (-364.1704, 144.8259) centre (-363.7436, 145.0864) ccw
  arc A573 (-363.4831, 145.5132) -> (-363.3268, 145.4693) centre (-363.3268, 145.7693) ccw
  line L358 (-363.3268, 145.4693) -> (-362.4264, 145.4693)
  line L359 (-362.4264, 145.4693) -> (-361.5261, 145.4693)
  arc A574 (-361.5261, 145.4693) -> (-361.3698, 145.5132) centre (-361.5261, 145.7693) ccw
  arc A575 (-360.6825, 144.8259) -> (-361.3698, 145.5132) centre (-361.1093, 145.0864) ccw
  arc A576 (-360.6825, 144.8259) -> (-360.7264, 144.6696) centre (-360.4264, 144.6696) ccw
  line L360 (-360.7264, 144.6696) -> (-360.7264, 143.9693)
  line L361 (-360.7264, 143.9693) -> (-360.7264, 143.2689)
  arc A577 (-360.7264, 143.2689) -> (-360.6825, 143.1126) centre (-360.4264, 143.2689) ccw
  arc A578 (-361.3698, 142.4254) -> (-360.6825, 143.1126) centre (-361.1093, 142.8521) ccw
  arc A579 (-361.3698, 142.4254) -> (-361.5261, 142.4693) centre (-361.526, 142.1696) ccw
  line L362 (-361.5261, 142.4693) -> (-362.4264, 142.4693)
  line L363 (-362.4264, 142.4693) -> (-363.3268, 142.4693)
  arc A580 (-363.3268, 142.4693) -> (-363.4831, 142.4254) centre (-363.3268, 142.1693) ccw
  circle A581 centre (-348.4564, 138.8893) radius 0.875
  circle A582 centre (-357.3464, 138.8893) radius 0.875
  circle A583 centre (-362.4264, 138.8893) radius 1.9939
  arc A584 (-383.2204, 143.1126) -> (-382.5331, 142.4254) centre (-382.7936, 142.8521) ccw
  arc A585 (-383.2204, 143.1126) -> (-383.1764, 143.2689) centre (-383.4764, 143.2689) ccw
  line L364 (-383.1764, 143.2689) -> (-383.1764, 143.9693)
  line L365 (-383.1764, 143.9693) -> (-383.1764, 144.6696)
  arc A586 (-383.1764, 144.6696) -> (-383.2204, 144.8259) centre (-383.4764, 144.6696) ccw
  arc A587 (-382.5331, 145.5132) -> (-383.2204, 144.8259) centre (-382.7936, 145.0864) ccw
  arc A588 (-382.5331, 145.5132) -> (-382.3768, 145.4693) centre (-382.3768, 145.7693) ccw
  line L366 (-382.3768, 145.4693) -> (-381.4764, 145.4693)
  line L367 (-381.4764, 145.4693) -> (-380.5761, 145.4693)
  arc A589 (-380.5761, 145.4693) -> (-380.4198, 145.5132) centre (-380.5761, 145.7693) ccw
  arc A590 (-379.7325, 144.8259) -> (-380.4198, 145.5132) centre (-380.1593, 145.0864) ccw
  arc A591 (-379.7325, 144.8259) -> (-379.7764, 144.6696) centre (-379.4764, 144.6696) ccw
  line L368 (-379.7764, 144.6696) -> (-379.7764, 143.9693)
  line L369 (-379.7764, 143.9693) -> (-379.7764, 143.2689)
  arc A592 (-379.7764, 143.2689) -> (-379.7325, 143.1126) centre (-379.4764, 143.2689) ccw
  arc A593 (-380.4198, 142.4254) -> (-379.7325, 143.1126) centre (-380.1593, 142.8521) ccw
  arc A594 (-380.4198, 142.4254) -> (-380.5761, 142.4693) centre (-380.576, 142.1696) ccw
  line L370 (-380.5761, 142.4693) -> (-381.4764, 142.4693)
  line L371 (-381.4764, 142.4693) -> (-382.3768, 142.4693)
  arc A595 (-382.3768, 142.4693) -> (-382.5331, 142.4254) centre (-382.3768, 142.1693) ccw
  circle A596 centre (-367.5064, 138.8893) radius 0.875
  circle A597 centre (-376.3964, 138.8893) radius 0.875
  circle A598 centre (-381.4764, 138.8893) radius 1.9939
  circle A599 centre (-345.9164, 133.8093) radius 1.5
  circle A600 centre (-358.6164, 136.3493) radius 1.5
  circle A601 centre (-364.9664, 133.8093) radius 1.5
  circle A602 centre (-377.6664, 136.3493) radius 1.5
  circle A603 centre (-384.0164, 133.8093) radius 1.5
  circle A604 centre (-393.0652, 157.9393) radius 0.875
  circle A605 centre (-398.1452, 157.9393) radius 1.9939
  circle A606 centre (-403.2252, 157.9393) radius 0.875
  circle A607 centre (-394.3352, 155.3993) radius 1.5
  circle A608 centre (-400.6852, 152.8593) radius 1.5
  circle A609 centre (-425.2914, 160.1618) radius 1.5
  circle A610 centre (-431.6414, 157.6218) radius 1.5
  circle A611 centre (-447.8339, 157.9393) radius 0.875
  circle A612 centre (-452.9139, 157.9393) radius 1.9939
  circle A613 centre (-457.9939, 157.9393) radius 0.875
  circle A614 centre (-449.1039, 155.3993) radius 1.5
  circle A615 centre (-455.4539, 152.8593) radius 1.5
  circle A616 centre (-438.6264, 148.4143) radius 1.1
  circle A617 centre (-386.5564, 138.8893) radius 0.875
  arc A618 (-411.376, 142.4254) -> (-410.6888, 143.1126) centre (-411.1155, 142.8521) ccw
  arc A619 (-411.376, 142.4254) -> (-411.5323, 142.4693) centre (-411.5323, 142.1696) ccw
  line L372 (-411.5323, 142.4693) -> (-412.4327, 142.4693)
  line L373 (-412.4327, 142.4693) -> (-413.3331, 142.4693)
  arc A620 (-413.3331, 142.4693) -> (-413.4894, 142.4254) centre (-413.3331, 142.1693) ccw
  arc A621 (-414.1766, 143.1126) -> (-413.4894, 142.4254) centre (-413.7499, 142.8521) ccw
  arc A622 (-414.1766, 143.1126) -> (-414.1327, 143.2689) centre (-414.4327, 143.2689) ccw
  line L374 (-414.1327, 143.2689) -> (-414.1327, 143.9693)
  line L375 (-414.1327, 143.9693) -> (-414.1327, 144.6696)
  arc A623 (-414.1327, 144.6696) -> (-414.1766, 144.8259) centre (-414.4327, 144.6696) ccw
  arc A624 (-413.4894, 145.5132) -> (-414.1766, 144.8259) centre (-413.7499, 145.0864) ccw
  arc A625 (-413.4894, 145.5132) -> (-413.3331, 145.4693) centre (-413.3331, 145.7693) ccw
  line L376 (-413.3331, 145.4693) -> (-412.4327, 145.4693)
  line L377 (-412.4327, 145.4693) -> (-411.5323, 145.4693)
  arc A626 (-411.5323, 145.4693) -> (-411.376, 145.5132) centre (-411.5324, 145.7693) ccw
  arc A627 (-410.6888, 144.8259) -> (-411.376, 145.5132) centre (-411.1155, 145.0864) ccw
  arc A628 (-410.6888, 144.8259) -> (-410.7327, 144.6696) centre (-410.4326, 144.6696) ccw
  line L378 (-410.7327, 144.6696) -> (-410.7327, 143.9693)
  line L379 (-410.7327, 143.9693) -> (-410.7327, 143.2689)
  arc A629 (-410.7327, 143.2689) -> (-410.6888, 143.1126) centre (-410.4326, 143.2689) ccw
  circle A630 centre (-407.3527, 138.8893) radius 0.875
  circle A631 centre (-412.4327, 138.8893) radius 1.9939
  circle A632 centre (-417.5127, 138.8893) radius 0.875
  circle A633 centre (-408.6227, 136.3493) radius 1.5
  circle A634 centre (-414.9727, 133.8093) radius 1.5
  arc A635 (-454.6579, 143.1126) -> (-453.9706, 142.4254) centre (-454.2311, 142.8521) ccw
  arc A636 (-454.6579, 143.1126) -> (-454.6139, 143.2689) centre (-454.9139, 143.2689) ccw
  line L380 (-454.6139, 143.2689) -> (-454.6139, 143.9693)
  line L381 (-454.6139, 143.9693) -> (-454.6139, 144.6696)
  arc A637 (-454.6139, 144.6696) -> (-454.6579, 144.8259) centre (-454.9139, 144.6696) ccw
  arc A638 (-453.9706, 145.5132) -> (-454.6579, 144.8259) centre (-454.2311, 145.0864) ccw
  arc A639 (-453.9706, 145.5132) -> (-453.8143, 145.4693) centre (-453.8143, 145.7693) ccw
  line L382 (-453.8143, 145.4693) -> (-452.9139, 145.4693)
  line L383 (-452.9139, 145.4693) -> (-452.0136, 145.4693)
  arc A640 (-452.0136, 145.4693) -> (-451.8573, 145.5132) centre (-452.0136, 145.7693) ccw
  arc A641 (-451.17, 144.8259) -> (-451.8573, 145.5132) centre (-451.5968, 145.0864) ccw
  arc A642 (-451.17, 144.8259) -> (-451.2139, 144.6696) centre (-450.9139, 144.6696) ccw
  line L384 (-451.2139, 144.6696) -> (-451.2139, 143.9693)
  line L385 (-451.2139, 143.9693) -> (-451.2139, 143.2689)
  arc A643 (-451.2139, 143.2689) -> (-451.17, 143.1126) centre (-450.9139, 143.2689) ccw
  arc A644 (-451.8573, 142.4254) -> (-451.17, 143.1126) centre (-451.5968, 142.8521) ccw
  arc A645 (-451.8573, 142.4254) -> (-452.0136, 142.4693) centre (-452.0135, 142.1696) ccw
  line L386 (-452.0136, 142.4693) -> (-452.9139, 142.4693)
  line L387 (-452.9139, 142.4693) -> (-453.8143, 142.4693)
  arc A646 (-453.8143, 142.4693) -> (-453.9706, 142.4254) centre (-453.8143, 142.1693) ccw
  circle A647 centre (-447.8339, 138.8893) radius 0.875
  circle A648 centre (-452.9139, 138.8893) radius 1.9939
  circle A649 centre (-457.9939, 138.8893) radius 0.875
  circle A650 centre (-449.1039, 136.3493) radius 1.5
  circle A651 centre (-455.4539, 133.8093) radius 1.5
  circle A652 centre (-462.4389, 129.3643) radius 1.1
  arc A653 (-161.3448, 123.3754) -> (-160.6575, 124.0626) centre (-161.0843, 123.8021) ccw
  arc A654 (-161.3448, 123.3754) -> (-161.5011, 123.4193) centre (-161.501, 123.1196) ccw
  line L388 (-161.5011, 123.4193) -> (-162.4014, 123.4193)
  line L389 (-162.4014, 123.4193) -> (-163.3018, 123.4193)
  arc A655 (-163.3018, 123.4193) -> (-163.4581, 123.3754) centre (-163.3018, 123.1193) ccw
  arc A656 (-164.1454, 124.0626) -> (-163.4581, 123.3754) centre (-163.7186, 123.8021) ccw
  arc A657 (-164.1454, 124.0626) -> (-164.1014, 124.2189) centre (-164.4014, 124.2189) ccw
  line L390 (-164.1014, 124.2189) -> (-164.1014, 124.9193)
  line L391 (-164.1014, 124.9193) -> (-164.1014, 125.6196)
  arc A658 (-164.1014, 125.6196) -> (-164.1454, 125.7759) centre (-164.4014, 125.6196) ccw
  arc A659 (-163.4581, 126.4632) -> (-164.1454, 125.7759) centre (-163.7186, 126.0364) ccw
  arc A660 (-163.4581, 126.4632) -> (-163.3018, 126.4193) centre (-163.3018, 126.7193) ccw
  line L392 (-163.3018, 126.4193) -> (-162.4014, 126.4193)
  line L393 (-162.4014, 126.4193) -> (-161.5011, 126.4193)
  arc A661 (-161.5011, 126.4193) -> (-161.3448, 126.4632) centre (-161.5011, 126.7193) ccw
  arc A662 (-160.6575, 125.7759) -> (-161.3448, 126.4632) centre (-161.0843, 126.0364) ccw
  arc A663 (-160.6575, 125.7759) -> (-160.7014, 125.6196) centre (-160.4014, 125.6196) ccw
  line L394 (-160.7014, 125.6196) -> (-160.7014, 124.9193)
  line L395 (-160.7014, 124.9193) -> (-160.7014, 124.2189)
  arc A664 (-160.7014, 124.2189) -> (-160.6575, 124.0626) centre (-160.4014, 124.2189) ccw
  arc A665 (-185.1573, 123.3754) -> (-184.47, 124.0626) centre (-184.8968, 123.8021) ccw
  arc A666 (-185.1573, 123.3754) -> (-185.3136, 123.4193) centre (-185.3135, 123.1196) ccw
  line L396 (-185.3136, 123.4193) -> (-186.2139, 123.4193)
  line L397 (-186.2139, 123.4193) -> (-187.1143, 123.4193)
  arc A667 (-187.1143, 123.4193) -> (-187.2706, 123.3754) centre (-187.1143, 123.1193) ccw
  arc A668 (-187.9579, 124.0626) -> (-187.2706, 123.3754) centre (-187.5311, 123.8021) ccw
  arc A669 (-187.9579, 124.0626) -> (-187.9139, 124.2189) centre (-188.2139, 124.2189) ccw
  line L398 (-187.9139, 124.2189) -> (-187.9139, 124.9193)
  line L399 (-187.9139, 124.9193) -> (-187.9139, 125.6196)
  arc A670 (-187.9139, 125.6196) -> (-187.9579, 125.7759) centre (-188.2139, 125.6196) ccw
  arc A671 (-187.2706, 126.4632) -> (-187.9579, 125.7759) centre (-187.5311, 126.0364) ccw
  arc A672 (-187.2706, 126.4632) -> (-187.1143, 126.4193) centre (-187.1143, 126.7193) ccw
  line L400 (-187.1143, 126.4193) -> (-186.2139, 126.4193)
  line L401 (-186.2139, 126.4193) -> (-185.3136, 126.4193)
  arc A673 (-185.3136, 126.4193) -> (-185.1573, 126.4632) centre (-185.3136, 126.7193) ccw
  arc A674 (-184.47, 125.7759) -> (-185.1573, 126.4632) centre (-184.8968, 126.0364) ccw
  arc A675 (-184.47, 125.7759) -> (-184.5139, 125.6196) centre (-184.2139, 125.6196) ccw
  line L402 (-184.5139, 125.6196) -> (-184.5139, 124.9193)
  line L403 (-184.5139, 124.9193) -> (-184.5139, 124.2189)
  arc A676 (-184.5139, 124.2189) -> (-184.47, 124.0626) centre (-184.2139, 124.2189) ccw
  circle A677 centre (-157.3214, 119.8393) radius 0.875
  circle A678 centre (-162.4014, 119.8393) radius 1.9939
  circle A679 centre (-158.5914, 117.2993) radius 1.5
  circle A680 centre (-164.9414, 114.7593) radius 1.5
  circle A681 centre (-167.4814, 119.8393) radius 0.875
  circle A682 centre (-181.1339, 119.8393) radius 0.875
  circle A683 centre (-186.2139, 119.8393) radius 1.9939
  circle A684 centre (-182.4039, 117.2993) radius 1.5
  arc A685 (-204.2073, 123.3754) -> (-203.52, 124.0626) centre (-203.9468, 123.8021) ccw
  arc A686 (-204.2073, 123.3754) -> (-204.3636, 123.4193) centre (-204.3635, 123.1196) ccw
  line L404 (-204.3636, 123.4193) -> (-205.2639, 123.4193)
  line L405 (-205.2639, 123.4193) -> (-206.1643, 123.4193)
  arc A687 (-206.1643, 123.4193) -> (-206.3206, 123.3754) centre (-206.1643, 123.1193) ccw
  arc A688 (-207.0079, 124.0626) -> (-206.3206, 123.3754) centre (-206.5811, 123.8021) ccw
  arc A689 (-207.0079, 124.0626) -> (-206.9639, 124.2189) centre (-207.2639, 124.2189) ccw
  line L406 (-206.9639, 124.2189) -> (-206.9639, 124.9193)
  line L407 (-206.9639, 124.9193) -> (-206.9639, 125.6196)
  arc A690 (-206.9639, 125.6196) -> (-207.0079, 125.7759) centre (-207.2639, 125.6196) ccw